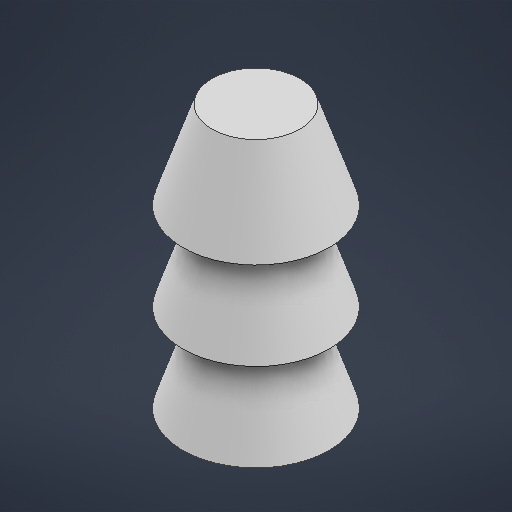
# Autodesk Inventor part: Valve_Plug_V2
Saved by Autodesk Inventor 2026.2 (Build 302298000, 298)
## iProperties
Created: 2026-01-25
Part Number: Valve_Plug_V2
Material: Generic
Document SubType Name: Modeling
Designer: vckot
Density: 1 g/cm^3
Appearance: Default
Author: vckot
Autodesk Inventor part; units mm, degrees
ref_plane "YZ Plane" through (0, 0, 0) normal (1, 0, 0) x (0, 1, 0)
ref_plane "XZ Plane" through (0, 0, 0) normal (0, 1, 0) x (-1, 0, 0)
ref_plane "XY Plane" through (0, 0, 0) normal (0, 0, 1) x (1, 0, 0)
sketch "Sketch1" plane through (0, 0, 0) normal (0, 0, 1) x (1, 0, 0)
  line L0 (-1.5, 0) -> (1.5, 0)
  line L1 (-2.5, -9) -> (2.5, -9)
  line L2 (-1.5, 0) -> (-2.5, -3)
  line L3 (1.5, 0) -> (2.5, -3)
  line L4 (-1.5, -3) -> (-1.5, -3)
  line L5 (1.5, -3) -> (1.5, -3)
  line L6 (-2.5, -6) -> (-1.5, -3)
  line L7 (1.5, -3) -> (2.5, -6)
  line L8 (-1.5, -6) -> (-1.5, -6)
  line L9 (1.5, -6) -> (1.5, -6)
  line L10 (-1.5, -6) -> (-2.5, -9)
  line L11 (1.5, -6) -> (2.5, -9)
  line L12 (0, 0) -> (0, -9)
  line L13 (-2.5, -6) -> (2.5, -6)
  line L14 (-2.5, -3) -> (2.5, -3)
  point P0 (0, -3)
  point P1 (0, -6)
  point P2 (0, -3)
  point P3 (0, -6)
  dimension "d1" = 5
  dimension "d5" = 5
  dimension "d15" = 5
  dimension "d16" = 1.5
  dimension "d17" = 1.5
  dimension "d18" = 1.5
  dimension "d19" = 1.5
  dimension "d20" = 3
  dimension "d21" = 3
  dimension "d22" = 3
  constraints: 30 end point, 6 point on line, 4 midpoint, 3 horizontal, 3 vertical alignment, 2 parallel, 1 equal length, 1 vertical
  measures "d1" distance of L2.end L3.end
  measures "d5" distance of L1.start L1.end
  measures "d15" distance of L6.start L7.end
  measures "d16" distance from line of L12 L9.start
  measures "d17" distance from line of L12 L8.start
  measures "d18" distance from line of L12 L5.start
  measures "d19" distance from line of L12 L4.start
  measures "d20" distance between parallel lines of L0 L14
  measures "d21" distance between parallel lines of L14 L13
  measures "d22" distance between parallel lines of L13 L1
revolve "Revolution1" add sketch "Sketch1" angle 360 about axis through (0, 0, 0) along (0, -1, 0) contours L0 L3 L14 L12 | L14 L7 L13 L12 | L13 L11 L1 L12
body "Solid1"
